Autodesk Inventor part; units mm, degrees
(part 4 of 6)
  circle A124 centre (-88.9, -304.8) radius 1.9939 projected
  circle A125 centre (-304.8, -44.45) radius 1.9939 projected
  circle A126 centre (-304.8, 0) radius 1.9939 projected
  line L431 (-258.6314, -105.0267) -> (-280.5432, -126.9386) projected
  line L432 (-280.5432, -126.9386) -> (-298.45, -109.0318) projected
  line L433 (-298.45, -109.0318) -> (-298.45, -101.0217) projected
  line L434 (-298.45, -101.0217) -> (-280.5432, -83.1149) projected
  line L435 (-280.5432, -83.1149) -> (-258.6314, -105.0267) projected
  line L436 (-233.1274, -79.5228) -> (-255.0393, -101.4346) projected
  line L437 (-255.0393, -101.4346) -> (-276.9511, -79.5228) projected
  line L438 (-276.9511, -79.5228) -> (-255.0393, -57.611) projected
  line L439 (-255.0393, -57.611) -> (-233.1274, -79.5228) projected
  line L440 (-178.5275, -83.1149) -> (-156.6157, -105.0267) projected
  line L441 (-156.6157, -105.0267) -> (-178.5275, -126.9386) projected
  line L442 (-178.5275, -126.9386) -> (-200.4393, -105.0267) projected
  line L443 (-200.4393, -105.0267) -> (-178.5275, -83.1149) projected
  line L444 (-153.0236, -108.6189) -> (-131.1117, -130.5307) projected
  line L445 (-131.1117, -130.5307) -> (-153.0236, -152.4425) projected
  line L446 (-153.0236, -152.4425) -> (-174.9354, -130.5307) projected
  line L447 (-174.9354, -130.5307) -> (-153.0236, -108.6189) projected
  line L448 (-76.5118, -134.1228) -> (-54.6, -156.0346) projected
  line L449 (-54.6, -156.0346) -> (-76.5118, -177.9464) projected
  line L450 (-76.5118, -177.9464) -> (-98.4236, -156.0346) projected
  line L451 (-98.4236, -156.0346) -> (-76.5118, -134.1228) projected
  line L452 (51.0079, -159.6267) -> (72.9197, -181.5385) projected
  line L453 (72.9197, -181.5385) -> (51.0079, -203.4504) projected
  line L454 (51.0079, -203.4504) -> (29.096, -181.5385) projected
  line L455 (29.096, -181.5385) -> (51.0079, -159.6267) projected
  line L456 (-51.0079, -152.4425) -> (-72.9197, -130.5307) projected
  line L457 (-72.9197, -130.5307) -> (-51.0079, -108.6189) projected
  line L458 (-51.0079, -108.6189) -> (-29.096, -130.5307) projected
  line L459 (-29.096, -130.5307) -> (-51.0079, -152.4425) projected
  line L460 (-146.05, -247.4846) -> (-146.05, -222.25) projected
  arc A127 (-146.05, -222.25) -> (-146.2009, -217.4573) centre (-222.25, -222.25) ccw projected
  line L461 (-146.2009, -217.4573) -> (-131.1117, -232.5464) projected
  line L462 (-131.1117, -232.5464) -> (-146.05, -247.4846) projected
  line L463 (-51.0079, -210.6346) -> (-29.096, -232.5464) projected
  line L464 (-29.096, -232.5464) -> (-51.0079, -254.4582) projected
  line L465 (-51.0079, -254.4582) -> (-72.9197, -232.5464) projected
  line L466 (-72.9197, -232.5464) -> (-51.0079, -210.6346) projected
  line L467 (-29.096, -283.5542) -> (-43.9918, -298.45) projected
  line L468 (-43.9918, -298.45) -> (-58.0239, -298.45) projected
  line L469 (-58.0239, -298.45) -> (-72.9197, -283.5542) projected
  line L470 (-72.9197, -283.5542) -> (-51.0079, -261.6424) projected
  line L471 (-51.0079, -261.6424) -> (-29.096, -283.5542) projected
  line L472 (-65.2081, -298.45) -> (-87.8154, -298.45) projected
  line L473 (-87.8154, -298.45) -> (-76.5118, -287.1463) projected
  line L474 (-76.5118, -287.1463) -> (-65.2081, -298.45) projected
  line L475 (94.9996, -298.45) -> (80.1039, -283.5542) projected
  line L476 (80.1039, -283.5542) -> (102.0157, -261.6424) projected
  line L477 (102.0157, -261.6424) -> (123.9275, -283.5542) projected
  line L478 (123.9275, -283.5542) -> (109.0318, -298.45) projected
  line L479 (109.0318, -298.45) -> (94.9996, -298.45) projected
  line L480 (36.8076, -298.45) -> (14.2003, -298.45) projected
  line L481 (14.2003, -298.45) -> (25.5039, -287.1463) projected
  line L482 (25.5039, -287.1463) -> (36.8076, -298.45) projected
  line L483 (102.0157, -203.4504) -> (80.1039, -181.5385) projected
  line L484 (80.1039, -181.5385) -> (102.0157, -159.6267) projected
  line L485 (102.0157, -159.6267) -> (123.9275, -181.5385) projected
  line L486 (123.9275, -181.5385) -> (102.0157, -203.4504) projected
  line L487 (204.0314, -57.611) -> (225.9432, -79.5228) projected
  line L488 (225.9432, -79.5228) -> (204.0314, -101.4346) projected
  line L489 (204.0314, -101.4346) -> (182.1196, -79.5228) projected
  line L490 (182.1196, -79.5228) -> (204.0314, -57.611) projected
  line L491 (284.1353, -28.515) -> (298.45, -14.2003) projected
  line L492 (298.45, -14.2003) -> (298.45, -42.8297) projected
  line L493 (298.45, -42.8297) -> (284.1353, -28.515) projected
  line L494 (280.5432, -75.9307) -> (258.6314, -54.0189) projected
  line L495 (258.6314, -54.0189) -> (280.5432, -32.1071) projected
  line L496 (280.5432, -32.1071) -> (298.45, -50.0139) projected
  line L497 (298.45, -50.0139) -> (298.45, -58.0239) projected
  line L498 (298.45, -58.0239) -> (280.5432, -75.9307) projected
  arc A128 (222.25, -146.05) -> (217.4573, -146.2009) centre (222.25, -222.25) ccw projected
  line L499 (217.4573, -146.2009) -> (229.5353, -134.1228) projected
  line L500 (229.5353, -134.1228) -> (241.4626, -146.05) projected
  line L501 (241.4626, -146.05) -> (222.25, -146.05) projected
  line L502 (149.4183, -199.8451) -> (131.1117, -181.5385) projected
  line L503 (131.1117, -181.5385) -> (153.0236, -159.6267) projected
  line L504 (153.0236, -159.6267) -> (165.1681, -171.7713) projected
  arc A129 (165.1681, -171.7713) -> (149.4183, -199.8451) centre (222.25, -222.25) ccw projected
  line L505 (21.9118, -283.5542) -> (7.0161, -298.45) projected
  line L506 (7.0161, -298.45) -> (-7.0161, -298.45) projected
  line L507 (-7.0161, -298.45) -> (-21.9118, -283.5542) projected
  line L508 (-21.9118, -283.5542) -> (0, -261.6424) projected
  line L509 (0, -261.6424) -> (21.9118, -283.5542) projected
  line L510 (284.1353, 124.5086) -> (298.45, 138.8233) projected
  line L511 (298.45, 138.8233) -> (298.45, 110.1939) projected
  line L512 (298.45, 110.1939) -> (284.1353, 124.5086) projected
  line L513 (280.5432, 77.0928) -> (258.6314, 99.0047) projected
  line L514 (258.6314, 99.0047) -> (280.5432, 120.9165) projected
  line L515 (280.5432, 120.9165) -> (298.45, 103.0097) projected
  line L516 (298.45, 103.0097) -> (298.45, 94.9996) projected
  line L517 (298.45, 94.9996) -> (280.5432, 77.0928) projected
  line L518 (255.0393, 0.5811) -> (233.1274, 22.4929) projected
  line L519 (233.1274, 22.4929) -> (255.0393, 44.4047) projected
  line L520 (255.0393, 44.4047) -> (276.9511, 22.4929) projected
  line L521 (276.9511, 22.4929) -> (255.0393, 0.5811) projected
  line L522 (229.5353, -24.9229) -> (207.6235, -3.011) projected
  line L523 (207.6235, -3.011) -> (229.5353, 18.9008) projected
  line L524 (229.5353, 18.9008) -> (251.4472, -3.011) projected
  line L525 (251.4472, -3.011) -> (229.5353, -24.9229) projected
  line L526 (153.0236, -6.6031) -> (174.9354, -28.515) projected
  line L527 (174.9354, -28.515) -> (153.0236, -50.4268) projected
  line L528 (153.0236, -50.4268) -> (131.1117, -28.515) projected
  line L529 (131.1117, -28.515) -> (153.0236, -6.6031) projected
  line L530 (174.933, 22.4952) -> (159.5933, 7.1508) projected
  line L531 (159.5933, 7.1508) -> (153.0236, 0.5811) projected
  line L532 (153.0236, 0.5811) -> (131.1117, 22.4929) projected
  line L533 (131.1117, 22.4929) -> (153.0236, 44.4047) projected
  line L534 (153.0236, 44.4047) -> (174.933, 22.4952) projected
  line L535 (127.5196, 69.9086) -> (149.4315, 47.9968) projected
  line L536 (149.4315, 47.9968) -> (127.5196, 26.085) projected
  line L537 (127.5196, 26.085) -> (105.6078, 47.9968) projected
  line L538 (105.6078, 47.9968) -> (127.5196, 69.9086) projected
  line L539 (178.5275, 77.0928) -> (156.6157, 99.0047) projected
  line L540 (156.6157, 99.0047) -> (178.5275, 120.9165) projected
  line L541 (178.5275, 120.9165) -> (200.4393, 99.0047) projected
  line L542 (200.4393, 99.0047) -> (178.5275, 77.0928) projected
  line L543 (102.0157, 153.6046) -> (80.1039, 175.5165) projected
  line L544 (80.1039, 175.5165) -> (102.0157, 197.4283) projected
  line L545 (102.0157, 197.4283) -> (123.9275, 175.5165) projected
  line L546 (123.9275, 175.5165) -> (102.0157, 153.6046) projected
  line L547 (-21.9118, 124.5086) -> (0, 146.4204) projected
  line L548 (0, 146.4204) -> (21.9118, 124.5086) projected
  line L549 (21.9118, 124.5086) -> (0, 102.5968) projected
  line L550 (0, 102.5968) -> (-21.9118, 124.5086) projected
  line L551 (146.05, 241.4626) -> (146.05, 222.25) projected
  arc A130 (146.05, 222.25) -> (146.9294, 210.7066) centre (222.25, 222.25) ccw projected
  line L552 (146.9294, 210.7066) -> (131.1117, 226.5243) projected
  line L553 (131.1117, 226.5243) -> (146.05, 241.4626) projected
  line L554 (102.0157, -152.4425) -> (80.1039, -130.5307) projected
  line L555 (80.1039, -130.5307) -> (102.0157, -108.6189) projected
  line L556 (102.0157, -108.6189) -> (123.9275, -130.5307) projected
  line L557 (123.9275, -130.5307) -> (102.0157, -152.4425) projected
  line L558 (25.5039, -134.1228) -> (47.4158, -156.0346) projected
  line L559 (47.4158, -156.0346) -> (25.5039, -177.9464) projected
  line L560 (25.5039, -177.9464) -> (3.5921, -156.0346) projected
  line L561 (3.5921, -156.0346) -> (25.5039, -134.1228) projected
  line L562 (76.5118, 273.9401) -> (98.4236, 252.0282) projected
  line L563 (98.4236, 252.0282) -> (76.5118, 230.1164) projected
  line L564 (76.5118, 230.1164) -> (54.6, 252.0282) projected
  line L565 (54.6, 252.0282) -> (76.5118, 273.9401) projected
  line L566 (25.5039, 230.1164) -> (3.5921, 252.0282) projected
  line L567 (3.5921, 252.0282) -> (25.5039, 273.9401) projected
  line L568 (25.5039, 273.9401) -> (47.4158, 252.0282) projected
  line L569 (47.4158, 252.0282) -> (25.5039, 230.1164) projected
  line L570 (-25.5039, 273.9401) -> (-3.5921, 252.0282) projected
  line L571 (-3.5921, 252.0282) -> (-25.5039, 230.1164) projected
  line L572 (-25.5039, 230.1164) -> (-47.4158, 252.0282) projected
  line L573 (-47.4158, 252.0282) -> (-25.5039, 273.9401) projected
  line L574 (-123.9275, 277.5322) -> (-103.0097, 298.45) projected
  line L575 (-103.0097, 298.45) -> (-101.0217, 298.45) projected
  line L576 (-101.0217, 298.45) -> (-80.1039, 277.5322) projected
  line L577 (-80.1039, 277.5322) -> (-102.0157, 255.6203) projected
  line L578 (-102.0157, 255.6203) -> (-123.9275, 277.5322) projected
  line L579 (-102.0157, 248.4361) -> (-80.1039, 226.5243) projected
  line L580 (-80.1039, 226.5243) -> (-102.0157, 204.6125) projected
  line L581 (-102.0157, 204.6125) -> (-123.9275, 226.5243) projected
  line L582 (-123.9275, 226.5243) -> (-102.0157, 248.4361) projected
  line L583 (-127.5196, 222.9322) -> (-105.6078, 201.0204) projected
  line L584 (-105.6078, 201.0204) -> (-127.5196, 179.1086) projected
  line L585 (-127.5196, 179.1086) -> (-149.1495, 200.7384) projected
  arc A131 (-149.1495, 200.7384) -> (-148.9209, 201.531) centre (-222.25, 222.25) ccw projected
  line L586 (-148.9209, 201.531) -> (-127.5196, 222.9322) projected
  line L587 (-102.0157, 197.4283) -> (-80.1039, 175.5165) projected
  line L588 (-80.1039, 175.5165) -> (-102.0157, 153.6046) projected
  line L589 (-102.0157, 153.6046) -> (-123.9275, 175.5165) projected
  line L590 (-123.9275, 175.5165) -> (-102.0157, 197.4283) projected
  line L591 (-25.5039, 171.9243) -> (-3.5921, 150.0125) projected
  line L592 (-3.5921, 150.0125) -> (-25.5039, 128.1007) projected
  line L593 (-25.5039, 128.1007) -> (-47.4158, 150.0125) projected
  line L594 (-47.4158, 150.0125) -> (-25.5039, 171.9243) projected
  line L595 (-153.0236, 146.4204) -> (-131.1117, 124.5086) projected
  line L596 (-131.1117, 124.5086) -> (-153.0236, 102.5968) projected
  line L597 (-153.0236, 102.5968) -> (-174.9354, 124.5086) projected
  line L598 (-174.9354, 124.5086) -> (-153.0236, 146.4204) projected
  line L599 (-153.0236, 95.4126) -> (-131.1117, 73.5007) projected
  line L600 (-131.1117, 73.5007) -> (-153.0236, 51.5889) projected
  line L601 (-153.0236, 51.5889) -> (-174.9354, 73.5007) projected
  line L602 (-174.9354, 73.5007) -> (-153.0236, 95.4126) projected
  line L603 (-127.5196, -75.9307) -> (-149.4315, -54.0189) projected
  line L604 (-149.4315, -54.0189) -> (-127.5196, -32.1071) projected
  line L605 (-127.5196, -32.1071) -> (-105.6078, -54.0189) projected
  line L606 (-105.6078, -54.0189) -> (-127.5196, -75.9307) projected
  line L607 (-153.0236, -57.611) -> (-131.1117, -79.5228) projected
  line L608 (-131.1117, -79.5228) -> (-153.0236, -101.4346) projected
  line L609 (-153.0236, -101.4346) -> (-174.9354, -79.5228) projected
  line L610 (-174.9354, -79.5228) -> (-153.0236, -57.611) projected
  arc A132 (-222.25, 146.05) -> (-210.7066, 146.9294) centre (-222.25, 222.25) ccw projected
  line L611 (-210.7066, 146.9294) -> (-229.5353, 128.1007) projected
  line L612 (-229.5353, 128.1007) -> (-247.4846, 146.05) projected
  line L613 (-247.4846, 146.05) -> (-222.25, 146.05) projected
  line L614 (-280.5432, 120.9165) -> (-258.6314, 99.0047) projected
  line L615 (-258.6314, 99.0047) -> (-280.5432, 77.0928) projected
  line L616 (-280.5432, 77.0928) -> (-298.45, 94.9996) projected
  line L617 (-298.45, 94.9996) -> (-298.45, 103.0097) projected
  line L618 (-298.45, 103.0097) -> (-280.5432, 120.9165) projected
  line L619 (-178.5275, 69.9086) -> (-156.6157, 47.9968) projected
  line L620 (-156.6157, 47.9968) -> (-178.5246, 26.0879) projected
  line L621 (-178.5246, 26.0879) -> (-200.4331, 48.0031) projected
  line L622 (-200.4331, 48.0031) -> (-178.5275, 69.9086) projected
  line L623 (-280.5432, 69.9086) -> (-258.6314, 47.9968) projected
  line L624 (-258.6314, 47.9968) -> (-280.5432, 26.085) projected
  line L625 (-280.5432, 26.085) -> (-298.45, 43.9918) projected
  line L626 (-298.45, 43.9918) -> (-298.45, 52.0018) projected
  line L627 (-298.45, 52.0018) -> (-280.5432, 69.9086) projected
  line L628 (-255.0393, -6.6031) -> (-233.1274, -28.515) projected
  line L629 (-233.1274, -28.515) -> (-255.0393, -50.4268) projected
  line L630 (-255.0393, -50.4268) -> (-276.9511, -28.515) projected
  line L631 (-276.9511, -28.515) -> (-255.0393, -6.6031) projected
  line L632 (-284.1353, -28.515) -> (-298.45, -42.8297) projected
  line L633 (-298.45, -42.8297) -> (-298.45, -14.2003) projected
  line L634 (-298.45, -14.2003) -> (-284.1353, -28.515) projected
  line L635 (-284.1353, -79.5228) -> (-298.45, -93.8375) projected
  line L636 (-298.45, -93.8375) -> (-298.45, -65.2081) projected
  line L637 (-298.45, -65.2081) -> (-284.1353, -79.5228) projected
  line L638 (-200.4393, -3.011) -> (-178.5275, 18.9008) projected
  line L639 (-178.5275, 18.9008) -> (-156.6157, -3.011) projected
  line L640 (-156.6157, -3.011) -> (-178.5275, -24.9229) projected
  line L641 (-178.5275, -24.9229) -> (-200.4393, -3.011) projected
  line L642 (-280.5432, 18.9008) -> (-258.6314, -3.011) projected
  line L643 (-258.6314, -3.011) -> (-280.5432, -24.9229) projected
  line L644 (-280.5432, -24.9229) -> (-298.45, -7.0161) projected
  line L645 (-298.45, -7.0161) -> (-298.45, 0.994) projected
  line L646 (-298.45, 0.994) -> (-280.5432, 18.9008) projected
  line L647 (-255.0393, 44.4047) -> (-233.1274, 22.4929) projected
  line L648 (-233.1274, 22.4929) -> (-255.0393, 0.5811) projected
  line L649 (-255.0393, 0.5811) -> (-276.9511, 22.4929) projected
  line L650 (-276.9511, 22.4929) -> (-255.0393, 44.4047) projected
  line L651 (-204.0314, 95.4126) -> (-182.1196, 73.5007) projected
  line L652 (-182.1196, 73.5007) -> (-204.0246, 51.5957) projected
  line L653 (-204.0246, 51.5957) -> (-225.9331, 73.5109) projected
  line L654 (-225.9331, 73.5109) -> (-204.0314, 95.4126) projected
  line L655 (-284.1353, 124.5086) -> (-298.45, 110.1939) projected
  line L656 (-298.45, 110.1939) -> (-298.45, 138.8233) projected
  line L657 (-298.45, 138.8233) -> (-284.1353, 124.5086) projected
  line L658 (0, 153.6046) -> (-21.9118, 175.5165) projected
  line L659 (-21.9118, 175.5165) -> (0, 197.4283) projected
  line L660 (0, 197.4283) -> (21.9118, 175.5165) projected
  line L661 (21.9118, 175.5165) -> (0, 153.6046) projected
  line L662 (-127.5196, -83.1149) -> (-105.6078, -105.0267) projected
  line L663 (-105.6078, -105.0267) -> (-127.5196, -126.9386) projected
  line L664 (-127.5196, -126.9386) -> (-149.4315, -105.0267) projected
  line L665 (-149.4315, -105.0267) -> (-127.5196, -83.1149) projected
  line L666 (-131.1117, -28.515) -> (-153.0236, -50.4268) projected
  line L667 (-153.0236, -50.4268) -> (-174.9354, -28.515) projected
  line L668 (-174.9354, -28.515) -> (-153.0236, -6.6031) projected
  line L669 (-153.0236, -6.6031) -> (-131.1117, -28.515) projected
  line L670 (-178.5275, 120.9165) -> (-156.6157, 99.0047) projected
  line L671 (-156.6157, 99.0047) -> (-178.5275, 77.0928) projected
  line L672 (-178.5275, 77.0928) -> (-200.4393, 99.0047) projected
  line L673 (-200.4393, 99.0047) -> (-178.5275, 120.9165) projected
  line L674 (-127.5196, 120.9165) -> (-105.6078, 99.0047) projected
  line L675 (-105.6078, 99.0047) -> (-127.5196, 77.0928) projected
  line L676 (-127.5196, 77.0928) -> (-149.4315, 99.0047) projected
  line L677 (-149.4315, 99.0047) -> (-127.5196, 120.9165) projected
  line L678 (-51.0079, 197.4283) -> (-29.096, 175.5165) projected
  line L679 (-29.096, 175.5165) -> (-51.0079, 153.6046) projected
  line L680 (-51.0079, 153.6046) -> (-72.9197, 175.5165) projected
  line L681 (-72.9197, 175.5165) -> (-51.0079, 197.4283) projected
  line L682 (-127.5196, 128.1007) -> (-149.4315, 150.0125) projected
  line L683 (-149.4315, 150.0125) -> (-127.5196, 171.9243) projected
  line L684 (-127.5196, 171.9243) -> (-105.6078, 150.0125) projected
  line L685 (-105.6078, 150.0125) -> (-127.5196, 128.1007) projected
  line L686 (-76.5118, 222.9322) -> (-54.6, 201.0204) projected
  line L687 (-54.6, 201.0204) -> (-76.5118, 179.1086) projected
  line L688 (-76.5118, 179.1086) -> (-98.4236, 201.0204) projected
  line L689 (-98.4236, 201.0204) -> (-76.5118, 222.9322) projected
  line L690 (-127.5196, 273.9401) -> (-105.6078, 252.0282) projected
  line L691 (-105.6078, 252.0282) -> (-127.5196, 230.1164) projected
  line L692 (-127.5196, 230.1164) -> (-146.05, 248.6468) projected
  line L693 (-146.05, 248.6468) -> (-146.05, 255.4097) projected
  line L694 (-146.05, 255.4097) -> (-127.5196, 273.9401) projected
  line L695 (-93.8375, 298.45) -> (-59.186, 298.45) projected
  line L696 (-59.186, 298.45) -> (-76.5118, 281.1243) projected
  line L697 (-76.5118, 281.1243) -> (-93.8375, 298.45) projected
  line L698 (0, 248.4361) -> (21.9118, 226.5243) projected
  line L699 (21.9118, 226.5243) -> (0, 204.6125) projected
  line L700 (0, 204.6125) -> (-21.9118, 226.5243) projected
  line L701 (-21.9118, 226.5243) -> (0, 248.4361) projected
  line L702 (51.0079, 204.6125) -> (29.096, 226.5243) projected
  line L703 (29.096, 226.5243) -> (51.0079, 248.4361) projected
  line L704 (51.0079, 248.4361) -> (72.9197, 226.5243) projected
  line L705 (72.9197, 226.5243) -> (51.0079, 204.6125) projected
  line L706 (101.0217, 298.45) -> (103.0097, 298.45) projected
  line L707 (103.0097, 298.45) -> (123.9275, 277.5322) projected
  line L708 (123.9275, 277.5322) -> (102.0157, 255.6203) projected
  line L709 (102.0157, 255.6203) -> (80.1039, 277.5322) projected
  line L710 (80.1039, 277.5322) -> (101.0217, 298.45) projected
  line L711 (51.0079, -152.4425) -> (29.096, -130.5307) projected
  line L712 (29.096, -130.5307) -> (51.0079, -108.6189) projected
  line L713 (51.0079, -108.6189) -> (72.9197, -130.5307) projected
  line L714 (72.9197, -130.5307) -> (51.0079, -152.4425) projected
  line L715 (127.5196, -126.9386) -> (105.6078, -105.0267) projected
  line L716 (105.6078, -105.0267) -> (127.5196, -83.1149) projected
  line L717 (127.5196, -83.1149) -> (149.4315, -105.0267) projected
  line L718 (149.4315, -105.0267) -> (127.5196, -126.9386) projected
  arc A133 (148.9209, 201.531) -> (149.1495, 200.7384) centre (222.25, 222.25) ccw projected
  line L719 (149.1495, 200.7384) -> (127.5196, 179.1086) projected
  line L720 (127.5196, 179.1086) -> (105.6078, 201.0204) projected
  line L721 (105.6078, 201.0204) -> (127.5196, 222.9322) projected
  line L722 (127.5196, 222.9322) -> (148.9209, 201.531) projected
  line L723 (25.5039, 128.1007) -> (3.5921, 150.0125) projected
  line L724 (3.5921, 150.0125) -> (25.5039, 171.9243) projected
  line L725 (25.5039, 171.9243) -> (47.4158, 150.0125) projected
  line L726 (47.4158, 150.0125) -> (25.5039, 128.1007) projected
  line L727 (127.5196, 128.1007) -> (105.6078, 150.0125) projected
  line L728 (105.6078, 150.0125) -> (127.5196, 171.9243) projected
  line L729 (127.5196, 171.9243) -> (149.4315, 150.0125) projected
  line L730 (149.4315, 150.0125) -> (127.5196, 128.1007) projected
  line L731 (102.0157, 102.5968) -> (80.1039, 124.5086) projected
  line L732 (80.1039, 124.5086) -> (102.0157, 146.4204) projected
  line L733 (102.0157, 146.4204) -> (123.9275, 124.5086) projected
  line L734 (123.9275, 124.5086) -> (102.0157, 102.5968) projected
  line L735 (153.0236, 51.5889) -> (131.1117, 73.5007) projected
  line L736 (131.1117, 73.5007) -> (153.0236, 95.4126) projected
  line L737 (153.0236, 95.4126) -> (174.9354, 73.5007) projected
  line L738 (174.9354, 73.5007) -> (153.0236, 51.5889) projected
  line L739 (153.0236, -57.611) -> (174.9354, -79.5228) projected
  line L740 (174.9354, -79.5228) -> (153.0236, -101.4346) projected
  line L741 (153.0236, -101.4346) -> (131.1117, -79.5228) projected
  line L742 (131.1117, -79.5228) -> (153.0236, -57.611) projected
  line L743 (178.5275, 18.9008) -> (200.4393, -3.011) projected
  line L744 (200.4393, -3.011) -> (178.5275, -24.9229) projected
  line L745 (178.5275, -24.9229) -> (156.6157, -3.011) projected
  line L746 (156.6157, -3.011) -> (178.5275, 18.9008) projected
  line L747 (178.5246, 26.0879) -> (156.6157, 47.9968) projected
  line L748 (156.6157, 47.9968) -> (178.5275, 69.9086) projected
  line L749 (178.5275, 69.9086) -> (200.4331, 48.0031) projected
  line L750 (200.4331, 48.0031) -> (178.5246, 26.0879) projected
  line L751 (280.5432, 26.085) -> (258.6314, 47.9968) projected
  line L752 (258.6314, 47.9968) -> (280.5432, 69.9086) projected
  line L753 (280.5432, 69.9086) -> (298.45, 52.0018) projected
  line L754 (298.45, 52.0018) -> (298.45, 43.9918) projected
  line L755 (298.45, 43.9918) -> (280.5432, 26.085) projected
  line L756 (233.1274, 124.5086) -> (254.6689, 146.05) projected
  line L757 (254.6689, 146.05) -> (255.4097, 146.05) projected
  line L758 (255.4097, 146.05) -> (276.9331, 124.5266) projected
  line L759 (276.9331, 124.5266) -> (255.0247, 102.6114) projected
  line L760 (255.0247, 102.6114) -> (233.1274, 124.5086) projected
  line L761 (284.1353, 73.5007) -> (298.45, 87.8154) projected
  line L762 (298.45, 87.8154) -> (298.45, 59.186) projected
  line L763 (298.45, 59.186) -> (284.1353, 73.5007) projected
  line L764 (102.0157, -210.6346) -> (123.9275, -232.5464) projected
  line L765 (123.9275, -232.5464) -> (102.0157, -254.4582) projected
  line L766 (102.0157, -254.4582) -> (80.1039, -232.5464) projected
  line L767 (80.1039, -232.5464) -> (102.0157, -210.6346) projected
  line L768 (168.6598, -168.0787) -> (156.6157, -156.0346) projected
  line L769 (156.6157, -156.0346) -> (178.5275, -134.1228) projected
  line L770 (178.5275, -134.1228) -> (195.3578, -150.9531) projected
  arc A134 (195.3578, -150.9531) -> (168.6598, -168.0787) centre (222.25, -222.25) ccw projected
  line L771 (292.4704, -146.05) -> (268.616, -146.05) projected
  line L772 (268.616, -146.05) -> (280.5432, -134.1228) projected
  line L773 (280.5432, -134.1228) -> (292.4704, -146.05) projected
  line L774 (298.45, -101.0217) -> (298.45, -109.0318) projected
  line L775 (298.45, -109.0318) -> (280.5432, -126.9386) projected
  line L776 (280.5432, -126.9386) -> (258.6314, -105.0267) projected
  line L777 (258.6314, -105.0267) -> (280.5432, -83.1149) projected
  line L778 (280.5432, -83.1149) -> (298.45, -101.0217) projected
  line L779 (280.5432, -24.9229) -> (258.6314, -3.011) projected
  line L780 (258.6314, -3.011) -> (280.5432, 18.9008) projected
  line L781 (280.5432, 18.9008) -> (298.45, 0.994) projected
  line L782 (298.45, 0.994) -> (298.45, -7.0161) projected
  line L783 (298.45, -7.0161) -> (280.5432, -24.9229) projected
  line L784 (178.5275, -83.1149) -> (200.4393, -105.0267) projected
  line L785 (200.4393, -105.0267) -> (178.5275, -126.9386) projected
  line L786 (178.5275, -126.9386) -> (156.6157, -105.0267) projected
  line L787 (156.6157, -105.0267) -> (178.5275, -83.1149) projected
  line L788 (76.5118, -185.1306) -> (98.4236, -207.0425) projected
  line L789 (98.4236, -207.0425) -> (76.5118, -228.9543) projected
  line L790 (76.5118, -228.9543) -> (54.6, -207.0425) projected
  line L791 (54.6, -207.0425) -> (76.5118, -185.1306) projected
  line L792 (72.9197, -283.5542) -> (58.0239, -298.45) projected
  line L793 (58.0239, -298.45) -> (43.9918, -298.45) projected
  line L794 (43.9918, -298.45) -> (29.096, -283.5542) projected
  line L795 (29.096, -283.5542) -> (51.0079, -261.6424) projected
  line L796 (51.0079, -261.6424) -> (72.9197, -283.5542) projected
  line L797 (146.05, -254.6689) -> (146.05, -261.4318) projected
  line L798 (146.05, -261.4318) -> (127.5196, -279.9621) projected
  line L799 (127.5196, -279.9621) -> (105.6078, -258.0503) projected
  line L800 (105.6078, -258.0503) -> (127.5196, -236.1385) projected
  line L801 (127.5196, -236.1385) -> (146.05, -254.6689) projected
  line L802 (-116.216, -298.45) -> (-138.8233, -298.45) projected
  line L803 (-138.8233, -298.45) -> (-127.5196, -287.1463) projected
  line L804 (-127.5196, -287.1463) -> (-116.216, -298.45) projected
  line L805 (-76.5118, -185.1306) -> (-54.6, -207.0425) projected
  line L806 (-54.6, -207.0425) -> (-76.5118, -228.9543) projected
  line L807 (-76.5118, -228.9543) -> (-98.4236, -207.0425) projected
  line L808 (-98.4236, -207.0425) -> (-76.5118, -185.1306) projected
  line L809 (-127.5196, -185.1306) -> (-105.6078, -207.0425) projected
  line L810 (-105.6078, -207.0425) -> (-127.5196, -228.9543) projected
  line L811 (-127.5196, -228.9543) -> (-147.1553, -209.3187) projected
  arc A135 (-147.1553, -209.3187) -> (-147.9092, -205.5202) centre (-222.25, -222.25) ccw projected
  line L812 (-147.9092, -205.5202) -> (-127.5196, -185.1306) projected
  line L813 (0, -152.4425) -> (-21.9118, -130.5307) projected
  line L814 (-21.9118, -130.5307) -> (0, -108.6189) projected
  line L815 (0, -108.6189) -> (21.9118, -130.5307) projected
  line L816 (21.9118, -130.5307) -> (0, -152.4425) projected
  line L817 (0, -254.4582) -> (-21.9118, -232.5464) projected
  line L818 (-21.9118, -232.5464) -> (0, -210.6346) projected
  line L819 (0, -210.6346) -> (21.9118, -232.5464) projected
  line L820 (21.9118, -232.5464) -> (0, -254.4582) projected
  line L821 (-102.0157, -108.6189) -> (-80.1039, -130.5307) projected
  line L822 (-80.1039, -130.5307) -> (-102.0157, -152.4425) projected
  line L823 (-102.0157, -152.4425) -> (-123.9275, -130.5307) projected
  line L824 (-123.9275, -130.5307) -> (-102.0157, -108.6189) projected
  arc A136 (-168.6598, -168.0787) -> (-195.3578, -150.9531) centre (-222.25, -222.25) ccw projected
  line L825 (-195.3578, -150.9531) -> (-178.5275, -134.1228) projected
  line L826 (-178.5275, -134.1228) -> (-156.6157, -156.0346) projected
  line L827 (-156.6157, -156.0346) -> (-168.6598, -168.0787) projected
  line L828 (-156.6157, -54.0189) -> (-178.5275, -75.9307) projected
  line L829 (-178.5275, -75.9307) -> (-200.4393, -54.0189) projected
  line L830 (-200.4393, -54.0189) -> (-178.5275, -32.1071) projected
  line L831 (-178.5275, -32.1071) -> (-156.6157, -54.0189) projected
  line L832 (-284.1353, -130.5307) -> (-298.45, -144.8454) projected
  line L833 (-298.45, -144.8454) -> (-298.45, -116.216) projected
  line L834 (-298.45, -116.216) -> (-284.1353, -130.5307) projected
  line L835 (-233.1274, -130.5307) -> (-248.6468, -146.05) projected
  line L836 (-248.6468, -146.05) -> (-261.4318, -146.05) projected
  line L837 (-261.4318, -146.05) -> (-276.9511, -130.5307) projected
  line L838 (-276.9511, -130.5307) -> (-255.0393, -108.6189) projected
  line L839 (-255.0393, -108.6189) -> (-233.1274, -130.5307) projected
  line L840 (-207.6235, -105.0267) -> (-229.5353, -126.9386) projected
  line L841 (-229.5353, -126.9386) -> (-251.4472, -105.0267) projected
  line L842 (-251.4472, -105.0267) -> (-229.5353, -83.1149) projected
  line L843 (-229.5353, -83.1149) -> (-207.6235, -105.0267) projected
  line L844 (-182.1196, -130.5307) -> (-200.7384, -149.1495) projected
  arc A137 (-200.7384, -149.1495) -> (-209.3187, -147.1553) centre (-222.25, -222.25) ccw projected
  line L845 (-209.3187, -147.1553) -> (-225.9432, -130.5307) projected
  line L846 (-225.9432, -130.5307) -> (-204.0314, -108.6189) projected
  line L847 (-204.0314, -108.6189) -> (-182.1196, -130.5307) projected
  line L848 (-127.5196, -134.1228) -> (-105.6078, -156.0346) projected
  line L849 (-105.6078, -156.0346) -> (-127.5196, -177.9464) projected
  line L850 (-127.5196, -177.9464) -> (-149.4315, -156.0346) projected
  line L851 (-149.4315, -156.0346) -> (-127.5196, -134.1228) projected
  line L852 (-51.0079, -159.6267) -> (-29.096, -181.5385) projected
  line L853 (-29.096, -181.5385) -> (-51.0079, -203.4504) projected
  line L854 (-51.0079, -203.4504) -> (-72.9197, -181.5385) projected
  line L855 (-72.9197, -181.5385) -> (-51.0079, -159.6267) projected
  line L856 (25.5039, -228.9543) -> (3.5921, -207.0425) projected
  line L857 (3.5921, -207.0425) -> (25.5039, -185.1306) projected
  line L858 (25.5039, -185.1306) -> (47.4158, -207.0425) projected
  line L859 (47.4158, -207.0425) -> (25.5039, -228.9543) projected
  line L860 (-25.5039, -177.9464) -> (-47.4158, -156.0346) projected
  line L861 (-47.4158, -156.0346) -> (-25.5039, -134.1228) projected
  line L862 (-25.5039, -134.1228) -> (-3.5921, -156.0346) projected
  line L863 (-3.5921, -156.0346) -> (-25.5039, -177.9464) projected
  line L864 (-146.05, -261.4318) -> (-146.05, -254.6689) projected
  line L865 (-146.05, -254.6689) -> (-127.5196, -236.1385) projected
  line L866 (-127.5196, -236.1385) -> (-105.6078, -258.0503) projected
  line L867 (-105.6078, -258.0503) -> (-127.5196, -279.9621) projected
  line L868 (-127.5196, -279.9621) -> (-146.05, -261.4318) projected
  line L869 (-76.5118, -236.1385) -> (-54.6, -258.0503) projected
  line L870 (-54.6, -258.0503) -> (-76.5118, -279.9621) projected
  line L871 (-76.5118, -279.9621) -> (-98.4236, -258.0503) projected
  line L872 (-98.4236, -258.0503) -> (-76.5118, -236.1385) projected
  line L873 (-109.0318, -298.45) -> (-123.9275, -283.5542) projected
  line L874 (-123.9275, -283.5542) -> (-102.0157, -261.6424) projected
  line L875 (-102.0157, -261.6424) -> (-80.1039, -283.5542) projected
  line L876 (-80.1039, -283.5542) -> (-94.9996, -298.45) projected
  line L877 (-94.9996, -298.45) -> (-109.0318, -298.45) projected
  line L878 (146.05, -268.616) -> (146.05, -298.45) projected
  line L879 (146.05, -298.45) -> (146.0075, -298.45) projected
  line L880 (146.0075, -298.45) -> (131.1117, -283.5542) projected
  line L881 (131.1117, -283.5542) -> (146.05, -268.616) projected
  line L882 (76.5118, -279.9621) -> (54.6, -258.0503) projected
  line L883 (54.6, -258.0503) -> (76.5118, -236.1385) projected
  line L884 (76.5118, -236.1385) -> (98.4236, -258.0503) projected
  line L885 (98.4236, -258.0503) -> (76.5118, -279.9621) projected
  line L886 (25.5039, -236.1385) -> (47.4158, -258.0503) projected
  line L887 (47.4158, -258.0503) -> (25.5039, -279.9621) projected
  line L888 (25.5039, -279.9621) -> (3.5921, -258.0503) projected
  line L889 (3.5921, -258.0503) -> (25.5039, -236.1385) projected
  line L890 (127.5196, -177.9464) -> (105.6078, -156.0346) projected
  line L891 (105.6078, -156.0346) -> (127.5196, -134.1228) projected
  line L892 (127.5196, -134.1228) -> (149.4315, -156.0346) projected
  line L893 (149.4315, -156.0346) -> (127.5196, -177.9464) projected
  line L894 (229.5353, -32.1071) -> (251.4472, -54.0189) projected
  line L895 (251.4472, -54.0189) -> (229.5353, -75.9307) projected
  line L896 (229.5353, -75.9307) -> (207.6235, -54.0189) projected
  line L897 (207.6235, -54.0189) -> (229.5353, -32.1071) projected
  line L898 (284.1353, -79.5228) -> (298.45, -65.2081) projected
  line L899 (298.45, -65.2081) -> (298.45, -93.8375) projected
  line L900 (298.45, -93.8375) -> (284.1353, -79.5228) projected
  line L901 (276.9511, -130.5307) -> (261.4318, -146.05) projected
  line L902 (261.4318, -146.05) -> (248.6468, -146.05) projected
  line L903 (248.6468, -146.05) -> (233.1274, -130.5307) projected
  line L904 (233.1274, -130.5307) -> (255.0393, -108.6189) projected
  line L905 (255.0393, -108.6189) -> (276.9511, -130.5307) projected
  line L906 (229.5353, -83.1149) -> (251.4472, -105.0267) projected
  line L907 (251.4472, -105.0267) -> (229.5353, -126.9386) projected
  line L908 (229.5353, -126.9386) -> (207.6235, -105.0267) projected
  line L909 (207.6235, -105.0267) -> (229.5353, -83.1149) projected
  arc A138 (146.2009, -217.4573) -> (146.05, -222.25) centre (222.25, -222.25) ccw projected
  line L910 (146.05, -222.25) -> (146.05, -247.4846) projected
  line L911 (146.05, -247.4846) -> (131.1117, -232.5464) projected
  line L912 (131.1117, -232.5464) -> (146.2009, -217.4573) projected
  line L913 (-14.2003, -298.45) -> (-36.8076, -298.45) projected
  line L914 (-36.8076, -298.45) -> (-25.5039, -287.1463) projected
  line L915 (-25.5039, -287.1463) -> (-14.2003, -298.45) projected
  line L916 (262.5939, 146.05) -> (298.45, 146.05) projected
  line L917 (298.45, 146.05) -> (280.5247, 128.1192) projected
  line L918 (280.5247, 128.1192) -> (262.5939, 146.05) projected
  line L919 (229.5246, 77.1035) -> (207.6235, 99.0047) projected
  line L920 (207.6235, 99.0047) -> (229.5353, 120.9165) projected
  line L921 (229.5353, 120.9165) -> (251.4331, 99.0187) projected
  line L922 (251.4331, 99.0187) -> (229.5246, 77.1035) projected
  line L923 (229.5353, 26.085) -> (207.6235, 47.9968) projected
  line L924 (207.6235, 47.9968) -> (229.5353, 69.9086) projected
  line L925 (229.5353, 69.9086) -> (251.4472, 47.9968) projected
  line L926 (251.4472, 47.9968) -> (229.5353, 26.085) projected
  line L927 (204.0314, -6.6031) -> (225.9432, -28.515) projected
  line L928 (225.9432, -28.515) -> (204.0314, -50.4268) projected
  line L929 (204.0314, -50.4268) -> (182.1196, -28.515) projected
  line L930 (182.1196, -28.515) -> (204.0314, -6.6031) projected
  line L931 (127.5196, -32.1071) -> (149.4315, -54.0189) projected
  line L932 (149.4315, -54.0189) -> (127.5196, -75.9307) projected
  line L933 (127.5196, -75.9307) -> (105.6078, -54.0189) projected
  line L934 (105.6078, -54.0189) -> (127.5196, -32.1071) projected
  line L935 (127.5196, 18.9008) -> (149.4315, -3.011) projected
  line L936 (149.4315, -3.011) -> (127.5196, -24.9229) projected
  line L937 (127.5196, -24.9229) -> (105.6078, -3.011) projected
  line L938 (105.6078, -3.011) -> (127.5196, 18.9008) projected
  line L939 (204.0314, 102.5968) -> (182.1196, 124.5086) projected
  line L940 (182.1196, 124.5086) -> (204.0314, 146.4204) projected
  line L941 (204.0314, 146.4204) -> (225.9432, 124.5086) projected
  line L942 (225.9432, 124.5086) -> (204.0314, 102.5968) projected
  line L943 (51.0079, 146.4204) -> (72.9197, 124.5086) projected
  line L944 (72.9197, 124.5086) -> (51.0079, 102.5968) projected
  line L945 (51.0079, 102.5968) -> (29.096, 124.5086) projected
  line L946 (29.096, 124.5086) -> (51.0079, 146.4204) projected
  arc A139 (171.7713, 165.1681) -> (199.8451, 149.4183) centre (222.25, 222.25) ccw projected
  line L947 (199.8451, 149.4183) -> (178.5275, 128.1007) projected
  line L948 (178.5275, 128.1007) -> (156.6157, 150.0125) projected
  line L949 (156.6157, 150.0125) -> (171.7713, 165.1681) projected
  line L950 (76.5118, 128.1007) -> (54.6, 150.0125) projected
  line L951 (54.6, 150.0125) -> (76.5118, 171.9243) projected
  line L952 (76.5118, 171.9243) -> (98.4236, 150.0125) projected
  line L953 (98.4236, 150.0125) -> (76.5118, 128.1007) projected
  line L954 (54.6, 201.0204) -> (76.5118, 222.9322) projected
  line L955 (76.5118, 222.9322) -> (98.4236, 201.0204) projected
  line L956 (98.4236, 201.0204) -> (76.5118, 179.1086) projected
  line L957 (76.5118, 179.1086) -> (54.6, 201.0204) projected
  line L958 (105.6078, 252.0282) -> (127.5196, 273.9401) projected
  line L959 (127.5196, 273.9401) -> (146.05, 255.4097) projected
  line L960 (146.05, 255.4097) -> (146.05, 248.6468) projected
  line L961 (146.05, 248.6468) -> (127.5196, 230.1164) projected
  line L962 (127.5196, 230.1164) -> (105.6078, 252.0282) projected
  line L963 (131.1117, 277.5322) -> (146.05, 292.4704) projected
  line L964 (146.05, 292.4704) -> (146.05, 262.5939) projected
  line L965 (146.05, 262.5939) -> (131.1117, 277.5322) projected
  line L966 (52.0018, 298.45) -> (72.9197, 277.5322) projected
  line L967 (72.9197, 277.5322) -> (51.0079, 255.6203) projected
  line L968 (51.0079, 255.6203) -> (29.096, 277.5322) projected
  line L969 (29.096, 277.5322) -> (50.0139, 298.45) projected
  line L970 (50.0139, 298.45) -> (52.0018, 298.45) projected
  line L971 (-21.9118, 277.5322) -> (-0.994, 298.45) projected
  line L972 (-0.994, 298.45) -> (0.994, 298.45) projected
  line L973 (0.994, 298.45) -> (21.9118, 277.5322) projected
  line L974 (21.9118, 277.5322) -> (0, 255.6203) projected
  line L975 (0, 255.6203) -> (-21.9118, 277.5322) projected
  line L976 (-42.8297, 298.45) -> (-8.1782, 298.45) projected
  line L977 (-8.1782, 298.45) -> (-25.5039, 281.1243) projected
  line L978 (-25.5039, 281.1243) -> (-42.8297, 298.45) projected
  line L979 (-144.8454, 298.45) -> (-110.1939, 298.45) projected
  line L980 (-110.1939, 298.45) -> (-127.5196, 281.1243) projected
  line L981 (-127.5196, 281.1243) -> (-144.8454, 298.45) projected
  line L982 (-76.5118, 230.1164) -> (-98.4236, 252.0282) projected
  line L983 (-98.4236, 252.0282) -> (-76.5118, 273.9401) projected
  line L984 (-76.5118, 273.9401) -> (-54.6, 252.0282) projected
  line L985 (-54.6, 252.0282) -> (-76.5118, 230.1164) projected
  arc A140 (-146.9294, 210.7066) -> (-146.05, 222.25) centre (-222.25, 222.25) ccw projected
  line L986 (-146.05, 222.25) -> (-146.05, 241.4626) projected
  line L987 (-146.05, 241.4626) -> (-131.1117, 226.5243) projected
  line L988 (-131.1117, 226.5243) -> (-146.9294, 210.7066) projected
  line L989 (-102.0157, 102.5968) -> (-123.9275, 124.5086) projected
  line L990 (-123.9275, 124.5086) -> (-102.0157, 146.4204) projected
  line L991 (-102.0157, 146.4204) -> (-80.1039, 124.5086) projected
  line L992 (-80.1039, 124.5086) -> (-102.0157, 102.5968) projected
  line L993 (-72.9197, 124.5086) -> (-51.0079, 146.4204) projected
  line L994 (-51.0079, 146.4204) -> (-29.096, 124.5086) projected
  line L995 (-29.096, 124.5086) -> (-51.0079, 102.5968) projected
  line L996 (-51.0079, 102.5968) -> (-72.9197, 124.5086) projected
  line L997 (-171.7713, 165.1681) -> (-156.6157, 150.0125) projected
  line L998 (-156.6157, 150.0125) -> (-178.5275, 128.1007) projected
  line L999 (-178.5275, 128.1007) -> (-199.8451, 149.4183) projected
  arc A141 (-199.8451, 149.4183) -> (-171.7713, 165.1681) centre (-222.25, 222.25) ccw projected
  line L1000 (-149.4315, 47.9968) -> (-127.5196, 69.9086) projected
  line L1001 (-127.5196, 69.9086) -> (-105.6078, 47.9968) projected
  line L1002 (-105.6078, 47.9968) -> (-127.5196, 26.085) projected
  line L1003 (-127.5196, 26.085) -> (-149.4315, 47.9968) projected
  line L1004 (-105.6078, -3.011) -> (-127.5196, -24.9229) projected
  line L1005 (-127.5196, -24.9229) -> (-149.4315, -3.011) projected
  line L1006 (-149.4315, -3.011) -> (-127.5196, 18.9008) projected
  line L1007 (-127.5196, 18.9008) -> (-105.6078, -3.011) projected
  line L1008 (-25.5039, 179.1086) -> (-47.4158, 201.0204) projected
  line L1009 (-47.4158, 201.0204) -> (-25.5039, 222.9322) projected
  line L1010 (-25.5039, 222.9322) -> (-3.5921, 201.0204) projected
  line L1011 (-3.5921, 201.0204) -> (-25.5039, 179.1086) projected
  line L1012 (-254.6689, 146.05) -> (-233.1274, 124.5086) projected
  line L1013 (-233.1274, 124.5086) -> (-255.0247, 102.6114) projected
  line L1014 (-255.0247, 102.6114) -> (-276.9331, 124.5266) projected
  line L1015 (-276.9331, 124.5266) -> (-255.4097, 146.05) projected
  line L1016 (-255.4097, 146.05) -> (-254.6689, 146.05) projected
  line L1017 (-255.0393, 95.4126) -> (-233.1274, 73.5007) projected
  line L1018 (-233.1274, 73.5007) -> (-255.0393, 51.5889) projected
  line L1019 (-255.0393, 51.5889) -> (-276.9511, 73.5007) projected
  line L1020 (-276.9511, 73.5007) -> (-255.0393, 95.4126) projected
  line L1021 (-204.0314, 44.4047) -> (-182.1196, 22.4929) projected
  line L1022 (-182.1196, 22.4929) -> (-204.0314, 0.5811) projected
  line L1023 (-204.0314, 0.5811) -> (-225.9432, 22.4929) projected
  line L1024 (-225.9432, 22.4929) -> (-204.0314, 44.4047) projected
  line L1025 (-284.1353, 73.5007) -> (-298.45, 59.186) projected
  line L1026 (-298.45, 59.186) -> (-298.45, 87.8154) projected
  line L1027 (-298.45, 87.8154) -> (-284.1353, 73.5007) projected
  line L1028 (-229.5353, 18.9008) -> (-207.6235, -3.011) projected
  line L1029 (-207.6235, -3.011) -> (-229.5353, -24.9229) projected
  line L1030 (-229.5353, -24.9229) -> (-251.4472, -3.011) projected
  line L1031 (-251.4472, -3.011) -> (-229.5353, 18.9008) projected
  line L1032 (-251.4472, -54.0189) -> (-229.5353, -32.1071) projected
  line L1033 (-229.5353, -32.1071) -> (-207.6235, -54.0189) projected
  line L1034 (-207.6235, -54.0189) -> (-229.5353, -75.9307) projected
  line L1035 (-229.5353, -75.9307) -> (-251.4472, -54.0189) projected
  line L1036 (-280.5432, -32.1071) -> (-258.6314, -54.0189) projected
  line L1037 (-258.6314, -54.0189) -> (-280.5432, -75.9307) projected
  line L1038 (-280.5432, -75.9307) -> (-298.45, -58.0239) projected
  line L1039 (-298.45, -58.0239) -> (-298.45, -50.0139) projected
  line L1040 (-298.45, -50.0139) -> (-280.5432, -32.1071) projected
  line L1041 (-225.9432, -28.515) -> (-204.0314, -6.6031) projected
  line L1042 (-204.0314, -6.6031) -> (-182.1196, -28.515) projected
  line L1043 (-182.1196, -28.515) -> (-204.0314, -50.4268) projected
  line L1044 (-204.0314, -50.4268) -> (-225.9432, -28.515) projected
  line L1045 (-284.1353, 22.4929) -> (-298.45, 8.1782) projected
  line L1046 (-298.45, 8.1782) -> (-298.45, 36.8076) projected
  line L1047 (-298.45, 36.8076) -> (-284.1353, 22.4929) projected
  line L1048 (-229.5353, 69.9086) -> (-207.6235, 47.9968) projected
  line L1049 (-207.6235, 47.9968) -> (-229.5353, 26.085) projected
  line L1050 (-229.5353, 26.085) -> (-251.4472, 47.9968) projected
  line L1051 (-251.4472, 47.9968) -> (-229.5353, 69.9086) projected
  line L1052 (-229.5353, 120.9165) -> (-207.6235, 99.0047) projected
  line L1053 (-207.6235, 99.0047) -> (-229.5246, 77.1035) projected
  line L1054 (-229.5246, 77.1035) -> (-251.4331, 99.0187) projected
  line L1055 (-251.4331, 99.0187) -> (-229.5353, 120.9165) projected
  line L1056 (-298.45, 146.05) -> (-262.5939, 146.05) projected
  line L1057 (-262.5939, 146.05) -> (-280.5247, 128.1192) projected
  line L1058 (-280.5247, 128.1192) -> (-298.45, 146.05) projected
  line L1059 (3.5921, 201.0204) -> (25.5039, 222.9322) projected
  line L1060 (25.5039, 222.9322) -> (47.4158, 201.0204) projected
  line L1061 (47.4158, 201.0204) -> (25.5039, 179.1086) projected
  line L1062 (25.5039, 179.1086) -> (3.5921, 201.0204) projected
  line L1063 (-153.0236, 44.4047) -> (-131.1117, 22.4929) projected
  line L1064 (-131.1117, 22.4929) -> (-153.0236, 0.5811) projected
  line L1065 (-153.0236, 0.5811) -> (-159.5933, 7.1508) projected
  line L1066 (-159.5933, 7.1508) -> (-174.933, 22.4952) projected
  line L1067 (-174.933, 22.4952) -> (-153.0236, 44.4047) projected
  line L1068 (-204.0314, 146.4204) -> (-182.1196, 124.5086) projected
  line L1069 (-182.1196, 124.5086) -> (-204.0314, 102.5968) projected
  line L1070 (-204.0314, 102.5968) -> (-225.9432, 124.5086) projected
  line L1071 (-225.9432, 124.5086) -> (-204.0314, 146.4204) projected
  line L1072 (-76.5118, 171.9243) -> (-54.6, 150.0125) projected
  line L1073 (-54.6, 150.0125) -> (-76.5118, 128.1007) projected
  line L1074 (-76.5118, 128.1007) -> (-98.4236, 150.0125) projected
  line L1075 (-98.4236, 150.0125) -> (-76.5118, 171.9243) projected
  line L1076 (-153.0236, 153.6046) -> (-168.0787, 168.6598) projected
  arc A142 (-168.0787, 168.6598) -> (-150.9531, 195.3578) centre (-222.25, 222.25) ccw projected
  line L1077 (-150.9531, 195.3578) -> (-131.1117, 175.5165) projected
  line L1078 (-131.1117, 175.5165) -> (-153.0236, 153.6046) projected
  line L1079 (-51.0079, 204.6125) -> (-72.9197, 226.5243) projected
  line L1080 (-72.9197, 226.5243) -> (-51.0079, 248.4361) projected
  line L1081 (-51.0079, 248.4361) -> (-29.096, 226.5243) projected
  line L1082 (-29.096, 226.5243) -> (-51.0079, 204.6125) projected
  line L1083 (-131.1117, 277.5322) -> (-146.05, 262.5939) projected
  line L1084 (-146.05, 262.5939) -> (-146.05, 292.4704) projected
  line L1085 (-146.05, 292.4704) -> (-131.1117, 277.5322) projected
  line L1086 (-50.0139, 298.45) -> (-29.096, 277.5322) projected
  line L1087 (-29.096, 277.5322) -> (-51.0079, 255.6203) projected
  line L1088 (-51.0079, 255.6203) -> (-72.9197, 277.5322) projected
  line L1089 (-72.9197, 277.5322) -> (-52.0018, 298.45) projected
  line L1090 (-52.0018, 298.45) -> (-50.0139, 298.45) projected
  line L1091 (8.1782, 298.45) -> (42.8297, 298.45) projected
  line L1092 (42.8297, 298.45) -> (25.5039, 281.1243) projected
  line L1093 (25.5039, 281.1243) -> (8.1782, 298.45) projected
  line L1094 (59.186, 298.45) -> (93.8375, 298.45) projected
  line L1095 (93.8375, 298.45) -> (76.5118, 281.1243) projected
  line L1096 (76.5118, 281.1243) -> (59.186, 298.45) projected
  line L1097 (110.1939, 298.45) -> (144.8454, 298.45) projected
  line L1098 (144.8454, 298.45) -> (127.5196, 281.1243) projected
  line L1099 (127.5196, 281.1243) -> (110.1939, 298.45) projected
  line L1100 (76.5118, -177.9464) -> (54.6, -156.0346) projected
  line L1101 (54.6, -156.0346) -> (76.5118, -134.1228) projected
  line L1102 (76.5118, -134.1228) -> (98.4236, -156.0346) projected
  line L1103 (98.4236, -156.0346) -> (76.5118, -177.9464) projected
  line L1104 (102.0157, 248.4361) -> (123.9275, 226.5243) projected
  line L1105 (123.9275, 226.5243) -> (102.0157, 204.6125) projected
  line L1106 (102.0157, 204.6125) -> (80.1039, 226.5243) projected
  line L1107 (80.1039, 226.5243) -> (102.0157, 248.4361) projected
  line L1108 (29.096, 175.5165) -> (51.0079, 197.4283) projected
  line L1109 (51.0079, 197.4283) -> (72.9197, 175.5165) projected
  line L1110 (72.9197, 175.5165) -> (51.0079, 153.6046) projected
  line L1111 (51.0079, 153.6046) -> (29.096, 175.5165) projected
  arc A143 (150.9531, 195.3578) -> (168.0787, 168.6598) centre (222.25, 222.25) ccw projected
  line L1112 (168.0787, 168.6598) -> (153.0236, 153.6046) projected
  line L1113 (153.0236, 153.6046) -> (131.1117, 175.5165) projected
  line L1114 (131.1117, 175.5165) -> (150.9531, 195.3578) projected
  line L1115 (153.0236, 102.5968) -> (131.1117, 124.5086) projected
  line L1116 (131.1117, 124.5086) -> (153.0236, 146.4204) projected
  line L1117 (153.0236, 146.4204) -> (174.9354, 124.5086) projected
  line L1118 (174.9354, 124.5086) -> (153.0236, 102.5968) projected
  line L1119 (127.5196, 77.0928) -> (105.6078, 99.0047) projected
  line L1120 (105.6078, 99.0047) -> (127.5196, 120.9165) projected
  line L1121 (127.5196, 120.9165) -> (149.4315, 99.0047) projected
  line L1122 (149.4315, 99.0047) -> (127.5196, 77.0928) projected
  line L1123 (178.5275, -32.1071) -> (200.4393, -54.0189) projected
  line L1124 (200.4393, -54.0189) -> (178.5275, -75.9307) projected
  line L1125 (178.5275, -75.9307) -> (156.6157, -54.0189) projected
  line L1126 (156.6157, -54.0189) -> (178.5275, -32.1071) projected
  line L1127 (204.0314, 0.5811) -> (182.1196, 22.4929) projected
  line L1128 (182.1196, 22.4929) -> (204.0314, 44.4047) projected
  line L1129 (204.0314, 44.4047) -> (225.9432, 22.4929) projected
  line L1130 (225.9432, 22.4929) -> (204.0314, 0.5811) projected
  line L1131 (204.0246, 51.5957) -> (182.1196, 73.5007) projected
  line L1132 (182.1196, 73.5007) -> (204.0314, 95.4126) projected
  line L1133 (204.0314, 95.4126) -> (225.9331, 73.5109) projected
  line L1134 (225.9331, 73.5109) -> (204.0246, 51.5957) projected
  line L1135 (255.0393, 51.5889) -> (233.1274, 73.5007) projected
  line L1136 (233.1274, 73.5007) -> (255.0393, 95.4126) projected
  line L1137 (255.0393, 95.4126) -> (276.9511, 73.5007) projected
  line L1138 (276.9511, 73.5007) -> (255.0393, 51.5889) projected
  line L1139 (222.25, 146.05) -> (247.4846, 146.05) projected
  line L1140 (247.4846, 146.05) -> (229.5353, 128.1007) projected
  line L1141 (229.5353, 128.1007) -> (210.7066, 146.9294) projected
  arc A144 (210.7066, 146.9294) -> (222.25, 146.05) centre (222.25, 222.25) ccw projected
  line L1142 (284.1353, 22.4929) -> (298.45, 36.8076) projected
  line L1143 (298.45, 36.8076) -> (298.45, 8.1782) projected
  line L1144 (298.45, 8.1782) -> (284.1353, 22.4929) projected
  line L1145 (127.5196, -228.9543) -> (105.6078, -207.0425) projected
  line L1146 (105.6078, -207.0425) -> (127.5196, -185.1306) projected
  line L1147 (127.5196, -185.1306) -> (147.9092, -205.5202) projected
  arc A145 (147.9092, -205.5202) -> (147.1553, -209.3187) centre (222.25, -222.25) ccw projected
  line L1148 (147.1553, -209.3187) -> (127.5196, -228.9543) projected
  line L1149 (225.9432, -130.5307) -> (209.3187, -147.1553) projected
  arc A146 (209.3187, -147.1553) -> (200.7384, -149.1495) centre (222.25, -222.25) ccw projected
  line L1150 (200.7384, -149.1495) -> (182.1196, -130.5307) projected
  line L1151 (182.1196, -130.5307) -> (204.0314, -108.6189) projected
  line L1152 (204.0314, -108.6189) -> (225.9432, -130.5307) projected
  line L1153 (255.0393, -57.611) -> (276.9511, -79.5228) projected
  line L1154 (276.9511, -79.5228) -> (255.0393, -101.4346) projected
  line L1155 (255.0393, -101.4346) -> (233.1274, -79.5228) projected
  line L1156 (233.1274, -79.5228) -> (255.0393, -57.611) projected
  line L1157 (284.1353, -130.5307) -> (298.45, -116.216) projected
  line L1158 (298.45, -116.216) -> (298.45, -144.8454) projected
  line L1159 (298.45, -144.8454) -> (284.1353, -130.5307) projected
  line L1160 (255.0393, -50.4268) -> (233.1274, -28.515) projected
  line L1161 (233.1274, -28.515) -> (255.0393, -6.6031) projected
  line L1162 (255.0393, -6.6031) -> (276.9511, -28.515) projected
  line L1163 (276.9511, -28.515) -> (255.0393, -50.4268) projected
  line L1164 (153.0236, -152.4425) -> (131.1117, -130.5307) projected
  line L1165 (131.1117, -130.5307) -> (153.0236, -108.6189) projected
  line L1166 (153.0236, -108.6189) -> (174.9354, -130.5307) projected
  line L1167 (174.9354, -130.5307) -> (153.0236, -152.4425) projected
  line L1168 (51.0079, -254.4582) -> (29.096, -232.5464) projected
  line L1169 (29.096, -232.5464) -> (51.0079, -210.6346) projected
  line L1170 (51.0079, -210.6346) -> (72.9197, -232.5464) projected
  line L1171 (72.9197, -232.5464) -> (51.0079, -254.4582) projected
  line L1172 (87.8154, -298.45) -> (65.2081, -298.45) projected
  line L1173 (65.2081, -298.45) -> (76.5118, -287.1463) projected
  line L1174 (76.5118, -287.1463) -> (87.8154, -298.45) projected
  line L1175 (138.8233, -298.45) -> (116.216, -298.45) projected
  line L1176 (116.216, -298.45) -> (127.5196, -287.1463) projected
  line L1177 (127.5196, -287.1463) -> (138.8233, -298.45) projected
  line L1178 (-146.0075, -298.45) -> (-146.05, -298.45) projected
  line L1179 (-146.05, -298.45) -> (-146.05, -268.616) projected
  line L1180 (-146.05, -268.616) -> (-131.1117, -283.5542) projected
  line L1181 (-131.1117, -283.5542) -> (-146.0075, -298.45) projected
  line L1182 (-25.5039, -236.1385) -> (-3.5921, -258.0503) projected
  line L1183 (-3.5921, -258.0503) -> (-25.5039, -279.9621) projected
  line L1184 (-25.5039, -279.9621) -> (-47.4158, -258.0503) projected
  line L1185 (-47.4158, -258.0503) -> (-25.5039, -236.1385) projected
  line L1186 (-102.0157, -210.6346) -> (-80.1039, -232.5464) projected
  line L1187 (-80.1039, -232.5464) -> (-102.0157, -254.4582) projected
  line L1188 (-102.0157, -254.4582) -> (-123.9275, -232.5464) projected
  line L1189 (-123.9275, -232.5464) -> (-102.0157, -210.6346) projected
  line L1190 (-102.0157, -159.6267) -> (-80.1039, -181.5385) projected
  line L1191 (-80.1039, -181.5385) -> (-102.0157, -203.4504) projected
  line L1192 (-102.0157, -203.4504) -> (-123.9275, -181.5385) projected
  line L1193 (-123.9275, -181.5385) -> (-102.0157, -159.6267) projected
  line L1194 (0, -203.4504) -> (-21.9118, -181.5385) projected
  line L1195 (-21.9118, -181.5385) -> (0, -159.6267) projected
  line L1196 (0, -159.6267) -> (21.9118, -181.5385) projected
  line L1197 (21.9118, -181.5385) -> (0, -203.4504) projected
  line L1198 (-25.5039, -185.1306) -> (-3.5921, -207.0425) projected
  line L1199 (-3.5921, -207.0425) -> (-25.5039, -228.9543) projected
  line L1200 (-25.5039, -228.9543) -> (-47.4158, -207.0425) projected
  line L1201 (-47.4158, -207.0425) -> (-25.5039, -185.1306) projected
  arc A147 (-149.4183, -199.8451) -> (-165.1681, -171.7713) centre (-222.25, -222.25) ccw projected
  line L1202 (-165.1681, -171.7713) -> (-153.0236, -159.6267) projected
  line L1203 (-153.0236, -159.6267) -> (-131.1117, -181.5385) projected
  line L1204 (-131.1117, -181.5385) -> (-149.4183, -199.8451) projected
  line L1205 (-222.25, -146.05) -> (-241.4626, -146.05) projected
  line L1206 (-241.4626, -146.05) -> (-229.5353, -134.1228) projected
  line L1207 (-229.5353, -134.1228) -> (-217.4573, -146.2009) projected
  arc A148 (-217.4573, -146.2009) -> (-222.25, -146.05) centre (-222.25, -222.25) ccw projected
  line L1208 (-182.1196, -79.5228) -> (-204.0314, -101.4346) projected
  line L1209 (-204.0314, -101.4346) -> (-225.9432, -79.5228) projected
  line L1210 (-225.9432, -79.5228) -> (-204.0314, -57.611) projected
  line L1211 (-204.0314, -57.611) -> (-182.1196, -79.5228) projected
  line L1212 (-268.616, -146.05) -> (-292.4704, -146.05) projected
  line L1213 (-292.4704, -146.05) -> (-280.5432, -134.1228) projected
  line L1214 (-280.5432, -134.1228) -> (-268.616, -146.05) projected
  line L1215 (-158.75, -311.15) -> (-158.75, -222.25) projected
  arc A149 (-158.75, -222.25) -> (-222.25, -158.75) centre (-222.25, -222.25) ccw projected
  line L1216 (-222.25, -158.75) -> (-311.15, -158.75) projected
  line L1217 (-311.15, 158.75) -> (-311.15, -158.75) projected
  line L1218 (-311.15, 158.75) -> (-222.25, 158.75) projected
  arc A150 (-222.25, 158.75) -> (-158.75, 222.25) centre (-222.25, 222.25) ccw projected
  line L1219 (-158.75, 222.25) -> (-158.75, 311.15) projected
  line L1220 (158.75, 311.15) -> (-158.75, 311.15) projected
  line L1221 (158.75, 311.15) -> (158.75, 222.25) projected
  arc A151 (158.75, 222.25) -> (222.25, 158.75) centre (222.25, 222.25) ccw projected
  line L1222 (222.25, 158.75) -> (311.15, 158.75) projected
  line L1223 (311.15, -158.75) -> (311.15, 158.75) projected
  line L1224 (311.15, -158.75) -> (222.25, -158.75) projected
  arc A152 (222.25, -158.75) -> (158.75, -222.25) centre (222.25, -222.25) ccw projected
  line L1225 (158.75, -222.25) -> (158.75, -311.15) projected
  line L1226 (-158.75, -311.15) -> (158.75, -311.15) projected
  circle A153 centre (-304.8, 88.9) radius 1.9939 projected
  circle A154 centre (-304.8, -133.35) radius 1.9939 projected
  circle A155 centre (0, -304.8) radius 1.9939 projected
  circle A156 centre (304.8, -133.35) radius 1.9939 projected
  circle A157 centre (304.8, 44.45) radius 1.9939 projected
  circle A158 centre (88.9, 304.8) radius 1.9939 projected
  circle A159 centre (-88.9, 304.8) radius 1.9939 projected
  circle A160 centre (-44.45, 304.8) radius 1.9939 projected
  circle A161 centre (133.35, 304.8) radius 1.9939 projected
  circle A162 centre (304.8, 0) radius 1.9939 projected
  circle A163 centre (133.35, -304.8) radius 1.9939 projected
  circle A164 centre (-44.45, -304.8) radius 1.9939 projected
  circle A165 centre (-304.8, -88.9) radius 1.9939 projected
  circle A166 centre (-304.8, 133.35) radius 1.9939 projected
  circle A167 centre (-304.8, 44.45) radius 1.9939 projected
  circle A168 centre (-133.35, -304.8) radius 1.9939 projected
  circle A169 centre (44.45, -304.8) radius 1.9939 projected
  circle A170 centre (304.8, -88.9) radius 1.9939 projected
  circle A171 centre (304.8, 88.9) radius 1.9939 projected
  circle A172 centre (44.45, 304.8) radius 1.9939 projected
  circle A173 centre (-133.35, 304.8) radius 1.9939 projected
  circle A174 centre (0, 304.8) radius 1.9939 projected
  circle A175 centre (304.8, 133.35) radius 1.9939 projected
  circle A176 centre (304.8, -44.45) radius 1.9939 projected
  circle A177 centre (88.9, -304.8) radius 1.9939 projected
  circle A178 centre (-88.9, -304.8) radius 1.9939 projected
  circle A179 centre (-304.8, -44.45) radius 1.9939 projected
  circle A180 centre (-304.8, 0) radius 1.9939 projected
  line L1227 (-280.5432, -126.9386) -> (-258.6314, -105.0267) projected
  line L1228 (-258.6314, -105.0267) -> (-280.5432, -83.1149) projected
  line L1229 (-280.5432, -83.1149) -> (-298.45, -101.0217) projected
  line L1230 (-298.45, -101.0217) -> (-298.45, -109.0318) projected
  line L1231 (-298.45, -109.0318) -> (-280.5432, -126.9386) projected
  line L1232 (-255.0393, -101.4346) -> (-233.1274, -79.5228) projected
  line L1233 (-233.1274, -79.5228) -> (-255.0393, -57.611) projected
  line L1234 (-255.0393, -57.611) -> (-276.9511, -79.5228) projected
  line L1235 (-276.9511, -79.5228) -> (-255.0393, -101.4346) projected
  line L1236 (-156.6157, -105.0267) -> (-178.5275, -83.1149) projected
  line L1237 (-178.5275, -83.1149) -> (-200.4393, -105.0267) projected
  line L1238 (-200.4393, -105.0267) -> (-178.5275, -126.9386) projected
  line L1239 (-178.5275, -126.9386) -> (-156.6157, -105.0267) projected
  line L1240 (-131.1117, -130.5307) -> (-153.0236, -108.6189) projected
  line L1241 (-153.0236, -108.6189) -> (-174.9354, -130.5307) projected
  line L1242 (-174.9354, -130.5307) -> (-153.0236, -152.4425) projected
  line L1243 (-153.0236, -152.4425) -> (-131.1117, -130.5307) projected
  line L1244 (-54.6, -156.0346) -> (-76.5118, -134.1228) projected